Autodesk Inventor part; units mm, degrees
(part 2 of 2)
sketch "Sketch6" plane through (0, 0, 0) normal (0, 0, -1) x (-1, 0, 0)
  line L0 (-4.3025, 26.9125) -> (-4.3025, 11.12) projected
  arc A0 (-4.3025, 26.9125) -> (-7.4775, 30.0875) centre (-7.4775, 26.9125) ccw projected
  line L1 (-8.7475, 30.0875) -> (-7.4775, 30.0875) projected
  arc A1 (-8.7475, 30.0875) -> (-11.9225, 26.9125) centre (-8.7475, 26.9125) ccw projected
  line L2 (-11.9225, 22.4675) -> (-11.9225, 26.9125) projected
  line L3 (-65.8975, 22.4675) -> (-11.9225, 22.4675) projected
  line L4 (-65.8975, 26.9125) -> (-65.8975, 22.4675) projected
  arc A2 (-65.8975, 26.9125) -> (-69.0725, 30.0875) centre (-69.0725, 26.9125) ccw projected
  line L5 (-70.3425, 30.0875) -> (-69.0725, 30.0875) projected
  arc A3 (-70.3425, 30.0875) -> (-73.5175, 26.9125) centre (-70.3425, 26.9125) ccw projected
  line L6 (-73.5175, 8.5836) -> (-73.5175, 26.9125) projected
  line L7 (-76.0575, 6.0436) -> (-73.5175, 8.5836) projected
  line L8 (-76.0575, -27.38) -> (-76.0575, 6.0436) projected
  line L9 (-76.1056, -27.9894) -> (-76.0575, -27.38) projected
  line L10 (-73.5175, -30.5776) -> (-76.1056, -27.9894) projected
  line L11 (-73.5175, -38.4925) -> (-73.5175, -30.5776) projected
  arc A4 (-73.5175, -38.4925) -> (-70.3425, -41.6675) centre (-70.3425, -38.4925) ccw projected
  line L12 (-69.0725, -41.6675) -> (-70.3425, -41.6675) projected
  arc A5 (-69.0725, -41.6675) -> (-65.8975, -38.4925) centre (-69.0725, -38.4925) ccw projected
  line L13 (-65.8975, -34.0475) -> (-65.8975, -38.4925) projected
  line L14 (-11.9225, -34.0475) -> (-65.8975, -34.0475) projected
  line L15 (-11.9225, -38.4925) -> (-11.9225, -34.0475) projected
  arc A6 (-11.9225, -38.4925) -> (-8.7475, -41.6675) centre (-8.7475, -38.4925) ccw projected
  line L16 (-7.4775, -41.6675) -> (-8.7475, -41.6675) projected
  arc A7 (-7.4775, -41.6675) -> (-4.3025, -38.4925) centre (-7.4775, -38.4925) ccw projected
  line L17 (-5.89, -20.285) -> (-5.89, 0) projected
  line L18 (-71.93, -32.46) -> (-5.89, -32.46) projected
  line L19 (-71.93, -29.92) -> (-71.93, -32.46) projected
  line L20 (-74.47, -27.38) -> (-71.93, -29.92) projected
  line L21 (-74.47, 5.386) -> (-74.47, -27.38) projected
  line L22 (-71.93, 7.926) -> (-74.47, 5.386) projected
  line L23 (-71.93, 20.88) -> (-71.93, 7.926) projected
  line L24 (-5.89, 20.88) -> (-71.93, 20.88) projected
  circle A8 centre (-8.1125, -37.8575) radius 2 projected
  circle A9 centre (-69.7075, -37.8575) radius 2 projected
  circle A10 centre (-69.7075, 26.2775) radius 2 projected
  circle A11 centre (-8.1125, 26.2775) radius 2 projected
  line L25 (-23.416, 17.135) -> (-48.816, 17.135) projected
  line L26 (-23.416, 19.545) -> (-23.416, 17.135) projected
  line L27 (-48.816, 19.545) -> (-23.416, 19.545) projected
  line L28 (-48.816, 17.135) -> (-48.816, 19.545) projected
  line L29 (-46.546, 17.34) -> (-46.546, 19.34) projected
  line L30 (-48.546, 17.34) -> (-46.546, 17.34) projected
  line L31 (-48.546, 19.34) -> (-48.546, 17.34) projected
  line L32 (-46.546, 19.34) -> (-48.546, 19.34) projected
  line L33 (-44.006, 17.34) -> (-44.006, 19.34) projected
  line L34 (-46.006, 17.34) -> (-44.006, 17.34) projected
  line L35 (-46.006, 19.34) -> (-46.006, 17.34) projected
  line L36 (-44.006, 19.34) -> (-46.006, 19.34) projected
  line L37 (-41.466, 17.34) -> (-41.466, 19.34) projected
  line L38 (-43.466, 17.34) -> (-41.466, 17.34) projected
  line L39 (-43.466, 19.34) -> (-43.466, 17.34) projected
  line L40 (-41.466, 19.34) -> (-43.466, 19.34) projected
  line L41 (-38.926, 17.34) -> (-38.926, 19.34) projected
  line L42 (-40.926, 17.34) -> (-38.926, 17.34) projected
  line L43 (-40.926, 19.34) -> (-40.926, 17.34) projected
  line L44 (-38.926, 19.34) -> (-40.926, 19.34) projected
  line L45 (-36.386, 17.34) -> (-36.386, 19.34) projected
  line L46 (-38.386, 17.34) -> (-36.386, 17.34) projected
  line L47 (-38.386, 19.34) -> (-38.386, 17.34) projected
  line L48 (-36.386, 19.34) -> (-38.386, 19.34) projected
  line L49 (-33.846, 17.34) -> (-33.846, 19.34) projected
  line L50 (-35.846, 17.34) -> (-33.846, 17.34) projected
  line L51 (-35.846, 19.34) -> (-35.846, 17.34) projected
  line L52 (-33.846, 19.34) -> (-35.846, 19.34) projected
  line L53 (-31.306, 17.34) -> (-31.306, 19.34) projected
  line L54 (-33.306, 17.34) -> (-31.306, 17.34) projected
  line L55 (-33.306, 19.34) -> (-33.306, 17.34) projected
  line L56 (-31.306, 19.34) -> (-33.306, 19.34) projected
  line L57 (-28.766, 17.34) -> (-28.766, 19.34) projected
  line L58 (-30.766, 17.34) -> (-28.766, 17.34) projected
  line L59 (-30.766, 19.34) -> (-30.766, 17.34) projected
  line L60 (-28.766, 19.34) -> (-30.766, 19.34) projected
  line L61 (-28.226, 17.34) -> (-26.226, 17.34) projected
  line L62 (-28.226, 19.34) -> (-28.226, 17.34) projected
  line L63 (-26.226, 19.34) -> (-28.226, 19.34) projected
  line L64 (-26.226, 17.34) -> (-26.226, 19.34) projected
  line L65 (-25.686, 19.34) -> (-25.686, 17.34) projected
  line L66 (-23.686, 19.34) -> (-25.686, 19.34) projected
  line L67 (-23.686, 17.34) -> (-23.686, 19.34) projected
  line L68 (-25.686, 17.34) -> (-23.686, 17.34) projected
  line L69 (-22.41, 16.27) -> (-20.87, 16.27) projected
  arc A12 (-22.41, 16.27) -> (-22.91, 15.77) centre (-22.41, 15.77) ccw projected
  arc A13 (-22.91, 15.77) -> (-23.41, 16.27) centre (-23.41, 15.77) ccw projected
  line L70 (-24.95, 16.27) -> (-23.41, 16.27) projected
  arc A14 (-24.95, 16.27) -> (-25.45, 15.77) centre (-24.95, 15.77) ccw projected
  arc A15 (-25.45, 15.77) -> (-25.95, 16.27) centre (-25.95, 15.77) ccw projected
  line L71 (-27.49, 16.27) -> (-25.95, 16.27) projected
  arc A16 (-27.49, 16.27) -> (-27.99, 15.77) centre (-27.49, 15.77) ccw projected
  line L72 (-27.99, 11.77) -> (-27.99, 15.77) projected
  arc A17 (-27.99, 11.77) -> (-27.49, 11.27) centre (-27.49, 11.77) ccw projected
  line L73 (-25.95, 11.27) -> (-27.49, 11.27) projected
  arc A18 (-25.95, 11.27) -> (-25.45, 11.77) centre (-25.95, 11.77) ccw projected
  arc A19 (-25.45, 11.77) -> (-24.95, 11.27) centre (-24.95, 11.77) ccw projected
  line L74 (-23.41, 11.27) -> (-24.95, 11.27) projected
  arc A20 (-23.41, 11.27) -> (-22.91, 11.77) centre (-23.41, 11.77) ccw projected
  arc A21 (-22.91, 11.77) -> (-22.41, 11.27) centre (-22.41, 11.77) ccw projected
  line L75 (-20.87, 11.27) -> (-22.41, 11.27) projected
  arc A22 (-20.87, 11.27) -> (-20.37, 11.77) centre (-20.87, 11.77) ccw projected
  line L76 (-20.37, 15.77) -> (-20.37, 11.77) projected
  arc A23 (-20.37, 15.77) -> (-20.87, 16.27) centre (-20.87, 15.77) ccw projected
  arc A24 (-24.555, 12.6317) -> (-24.555, 12.3643) centre (-24.178, 12.498) ccw projected
  line L77 (-24.555, 12.875) -> (-24.555, 12.6317) projected
  line L78 (-24.3117, 12.875) -> (-24.555, 12.875) projected
  arc A25 (-24.0443, 12.875) -> (-24.3117, 12.875) centre (-24.178, 12.498) ccw projected
  line L79 (-23.805, 12.875) -> (-24.0443, 12.875) projected
  line L80 (-23.805, 12.6425) -> (-23.805, 12.875) projected
  arc A26 (-23.805, 12.3535) -> (-23.805, 12.6425) centre (-24.178, 12.498) ccw projected
  line L81 (-23.805, 12.125) -> (-23.805, 12.3535) projected
  line L82 (-24.0335, 12.125) -> (-23.805, 12.125) projected
  arc A27 (-24.3225, 12.125) -> (-24.0335, 12.125) centre (-24.178, 12.498) ccw projected
  line L83 (-24.555, 12.125) -> (-24.3225, 12.125) projected
  line L84 (-24.555, 12.3643) -> (-24.555, 12.125) projected
  arc A28 (-24.555, 15.1717) -> (-24.555, 14.9043) centre (-24.178, 15.038) ccw projected
  line L85 (-24.555, 15.415) -> (-24.555, 15.1717) projected
  line L86 (-24.3117, 15.415) -> (-24.555, 15.415) projected
  arc A29 (-24.0443, 15.415) -> (-24.3117, 15.415) centre (-24.178, 15.038) ccw projected
  line L87 (-23.805, 15.415) -> (-24.0443, 15.415) projected
  line L88 (-23.805, 15.1825) -> (-23.805, 15.415) projected
  arc A30 (-23.805, 14.8935) -> (-23.805, 15.1825) centre (-24.178, 15.038) ccw projected
  line L89 (-23.805, 14.665) -> (-23.805, 14.8935) projected
  line L90 (-24.0335, 14.665) -> (-23.805, 14.665) projected
  arc A31 (-24.3225, 14.665) -> (-24.0335, 14.665) centre (-24.178, 15.038) ccw projected
  line L91 (-24.555, 14.665) -> (-24.3225, 14.665) projected
  line L92 (-24.555, 14.9043) -> (-24.555, 14.665) projected
  arc A32 (-27.095, 12.6317) -> (-27.095, 12.3643) centre (-26.718, 12.498) ccw projected
  line L93 (-27.095, 12.875) -> (-27.095, 12.6317) projected
  line L94 (-26.8517, 12.875) -> (-27.095, 12.875) projected
  arc A33 (-26.5843, 12.875) -> (-26.8517, 12.875) centre (-26.718, 12.498) ccw projected
  line L95 (-26.345, 12.875) -> (-26.5843, 12.875) projected
  line L96 (-26.345, 12.6425) -> (-26.345, 12.875) projected
  arc A34 (-26.345, 12.3535) -> (-26.345, 12.6425) centre (-26.718, 12.498) ccw projected
  line L97 (-26.345, 12.125) -> (-26.345, 12.3535) projected
  line L98 (-26.5735, 12.125) -> (-26.345, 12.125) projected
  arc A35 (-26.8625, 12.125) -> (-26.5735, 12.125) centre (-26.718, 12.498) ccw projected
  line L99 (-27.095, 12.125) -> (-26.8625, 12.125) projected
  line L100 (-27.095, 12.3643) -> (-27.095, 12.125) projected
  arc A36 (-27.095, 15.1717) -> (-27.095, 14.9043) centre (-26.718, 15.038) ccw projected
  line L101 (-27.095, 15.415) -> (-27.095, 15.1717) projected
  line L102 (-26.8517, 15.415) -> (-27.095, 15.415) projected
  arc A37 (-26.5843, 15.415) -> (-26.8517, 15.415) centre (-26.718, 15.038) ccw projected
  line L103 (-26.345, 15.415) -> (-26.5843, 15.415) projected
  line L104 (-26.345, 15.1825) -> (-26.345, 15.415) projected
  arc A38 (-26.345, 14.8935) -> (-26.345, 15.1825) centre (-26.718, 15.038) ccw projected
  line L105 (-26.345, 14.665) -> (-26.345, 14.8935) projected
  line L106 (-26.5735, 14.665) -> (-26.345, 14.665) projected
  arc A39 (-26.8625, 14.665) -> (-26.5735, 14.665) centre (-26.718, 15.038) ccw projected
  line L107 (-27.095, 14.665) -> (-26.8625, 14.665) projected
  line L108 (-27.095, 14.9043) -> (-27.095, 14.665) projected
  arc A40 (-22.015, 12.6317) -> (-22.015, 12.3643) centre (-21.638, 12.498) ccw projected
  line L109 (-22.015, 12.875) -> (-22.015, 12.6317) projected
  line L110 (-21.7717, 12.875) -> (-22.015, 12.875) projected
  arc A41 (-21.5043, 12.875) -> (-21.7717, 12.875) centre (-21.638, 12.498) ccw projected
  line L111 (-21.265, 12.875) -> (-21.5043, 12.875) projected
  line L112 (-21.265, 12.6425) -> (-21.265, 12.875) projected
  arc A42 (-21.265, 12.3535) -> (-21.265, 12.6425) centre (-21.638, 12.498) ccw projected
  line L113 (-21.265, 12.125) -> (-21.265, 12.3535) projected
  line L114 (-21.4935, 12.125) -> (-21.265, 12.125) projected
  arc A43 (-21.7825, 12.125) -> (-21.4935, 12.125) centre (-21.638, 12.498) ccw projected
  line L115 (-22.015, 12.125) -> (-21.7825, 12.125) projected
  line L116 (-22.015, 12.3643) -> (-22.015, 12.125) projected
  arc A44 (-22.015, 15.1717) -> (-22.015, 14.9043) centre (-21.638, 15.038) ccw projected
  line L117 (-22.015, 15.415) -> (-22.015, 15.1717) projected
  line L118 (-21.7717, 15.415) -> (-22.015, 15.415) projected
  arc A45 (-21.5043, 15.415) -> (-21.7717, 15.415) centre (-21.638, 15.038) ccw projected
  line L119 (-21.265, 15.415) -> (-21.5043, 15.415) projected
  line L120 (-21.265, 15.1825) -> (-21.265, 15.415) projected
  arc A46 (-21.265, 14.8935) -> (-21.265, 15.1825) centre (-21.638, 15.038) ccw projected
  line L121 (-21.265, 14.665) -> (-21.265, 14.8935) projected
  line L122 (-21.4935, 14.665) -> (-21.265, 14.665) projected
  arc A47 (-21.7825, 14.665) -> (-21.4935, 14.665) centre (-21.638, 15.038) ccw projected
  line L123 (-22.015, 14.665) -> (-21.7825, 14.665) projected
  line L124 (-22.015, 14.9043) -> (-22.015, 14.665) projected
  line L125 (-50.34, 17.135) -> (-70.66, 17.135) projected
  line L126 (-50.34, 19.545) -> (-50.34, 17.135) projected
  line L127 (-70.66, 19.545) -> (-50.34, 19.545) projected
  line L128 (-70.66, 17.135) -> (-70.66, 19.545) projected
  line L129 (-68.39, 17.34) -> (-68.39, 19.34) projected
  line L130 (-70.39, 17.34) -> (-68.39, 17.34) projected
  line L131 (-70.39, 19.34) -> (-70.39, 17.34) projected
  line L132 (-68.39, 19.34) -> (-70.39, 19.34) projected
  line L133 (-65.85, 17.34) -> (-65.85, 19.34) projected
  line L134 (-67.85, 17.34) -> (-65.85, 17.34) projected
  line L135 (-67.85, 19.34) -> (-67.85, 17.34) projected
  line L136 (-65.85, 19.34) -> (-67.85, 19.34) projected
  line L137 (-63.31, 17.34) -> (-63.31, 19.34) projected
  line L138 (-65.31, 17.34) -> (-63.31, 17.34) projected
  line L139 (-65.31, 19.34) -> (-65.31, 17.34) projected
  line L140 (-63.31, 19.34) -> (-65.31, 19.34) projected
  line L141 (-60.77, 17.34) -> (-60.77, 19.34) projected
  line L142 (-62.77, 17.34) -> (-60.77, 17.34) projected
  line L143 (-62.77, 19.34) -> (-62.77, 17.34) projected
  line L144 (-60.77, 19.34) -> (-62.77, 19.34) projected
  line L145 (-58.23, 17.34) -> (-58.23, 19.34) projected
  line L146 (-60.23, 17.34) -> (-58.23, 17.34) projected
  line L147 (-60.23, 19.34) -> (-60.23, 17.34) projected
  line L148 (-58.23, 19.34) -> (-60.23, 19.34) projected
  line L149 (-55.69, 17.34) -> (-55.69, 19.34) projected
  line L150 (-57.69, 17.34) -> (-55.69, 17.34) projected
  line L151 (-57.69, 19.34) -> (-57.69, 17.34) projected
  line L152 (-55.69, 19.34) -> (-57.69, 19.34) projected
  line L153 (-55.15, 17.34) -> (-53.15, 17.34) projected
  line L154 (-55.15, 19.34) -> (-55.15, 17.34) projected
  line L155 (-53.15, 19.34) -> (-55.15, 19.34) projected
  line L156 (-53.15, 17.34) -> (-53.15, 19.34) projected
  line L157 (-52.61, 19.34) -> (-52.61, 17.34) projected
  line L158 (-50.61, 19.34) -> (-52.61, 19.34) projected
  line L159 (-50.61, 17.34) -> (-50.61, 19.34) projected
  line L160 (-52.61, 17.34) -> (-50.61, 17.34) projected
  line L161 (-73.3, -2.8) -> (-73.3, -1.26) projected
  arc A48 (-73.3, -2.8) -> (-72.8, -3.3) centre (-72.8, -2.8) ccw projected
  arc A49 (-72.8, -3.3) -> (-73.3, -3.8) centre (-72.8, -3.8) ccw projected
  line L162 (-73.3, -5.34) -> (-73.3, -3.8) projected
  arc A50 (-73.3, -5.34) -> (-72.8, -5.84) centre (-72.8, -5.34) ccw projected
  arc A51 (-72.8, -5.84) -> (-73.3, -6.34) centre (-72.8, -6.34) ccw projected
  line L163 (-73.3, -7.88) -> (-73.3, -6.34) projected
  arc A52 (-73.3, -7.88) -> (-72.8, -8.38) centre (-72.8, -7.88) ccw projected
  line L164 (-68.8, -8.38) -> (-72.8, -8.38) projected
  arc A53 (-68.8, -8.38) -> (-68.3, -7.88) centre (-68.8, -7.88) ccw projected
  line L165 (-68.3, -6.34) -> (-68.3, -7.88) projected
  arc A54 (-68.3, -6.34) -> (-68.8, -5.84) centre (-68.8, -6.34) ccw projected
  arc A55 (-68.8, -5.84) -> (-68.3, -5.34) centre (-68.8, -5.34) ccw projected
  line L166 (-68.3, -3.8) -> (-68.3, -5.34) projected
  arc A56 (-68.3, -3.8) -> (-68.8, -3.3) centre (-68.8, -3.8) ccw projected
  arc A57 (-68.8, -3.3) -> (-68.3, -2.8) centre (-68.8, -2.8) ccw projected
  line L167 (-68.3, -1.26) -> (-68.3, -2.8) projected
  arc A58 (-68.3, -1.26) -> (-68.8, -0.76) centre (-68.8, -1.26) ccw projected
  line L168 (-72.8, -0.76) -> (-68.8, -0.76) projected
  arc A59 (-72.8, -0.76) -> (-73.3, -1.26) centre (-72.8, -1.26) ccw projected
  arc A60 (-69.905, -4.4308) -> (-69.905, -4.7092) centre (-69.53, -4.57) ccw projected
  line L169 (-69.905, -4.195) -> (-69.905, -4.4308) projected
  line L170 (-69.6692, -4.195) -> (-69.905, -4.195) projected
  arc A61 (-69.3908, -4.195) -> (-69.6692, -4.195) centre (-69.53, -4.57) ccw projected
  line L171 (-69.155, -4.195) -> (-69.3908, -4.195) projected
  line L172 (-69.155, -4.4308) -> (-69.155, -4.195) projected
  arc A62 (-69.155, -4.7092) -> (-69.155, -4.4308) centre (-69.53, -4.57) ccw projected
  line L173 (-69.155, -4.945) -> (-69.155, -4.7092) projected
  line L174 (-69.3908, -4.945) -> (-69.155, -4.945) projected
  arc A63 (-69.6692, -4.945) -> (-69.3908, -4.945) centre (-69.53, -4.57) ccw projected
  line L175 (-69.905, -4.945) -> (-69.6692, -4.945) projected
  line L176 (-69.905, -4.7092) -> (-69.905, -4.945) projected
  arc A64 (-72.445, -4.4308) -> (-72.445, -4.7092) centre (-72.07, -4.57) ccw projected
  line L177 (-72.445, -4.195) -> (-72.445, -4.4308) projected
  line L178 (-72.2092, -4.195) -> (-72.445, -4.195) projected
  arc A65 (-71.9308, -4.195) -> (-72.2092, -4.195) centre (-72.07, -4.57) ccw projected
  line L179 (-71.695, -4.195) -> (-71.9308, -4.195) projected
  line L180 (-71.695, -4.4308) -> (-71.695, -4.195) projected
  arc A66 (-71.695, -4.7092) -> (-71.695, -4.4308) centre (-72.07, -4.57) ccw projected
  line L181 (-71.695, -4.945) -> (-71.695, -4.7092) projected
  line L182 (-71.9308, -4.945) -> (-71.695, -4.945) projected
  arc A67 (-72.2092, -4.945) -> (-71.9308, -4.945) centre (-72.07, -4.57) ccw projected
  line L183 (-72.445, -4.945) -> (-72.2092, -4.945) projected
  line L184 (-72.445, -4.7092) -> (-72.445, -4.945) projected
  arc A68 (-69.905, -6.9708) -> (-69.905, -7.2492) centre (-69.53, -7.11) ccw projected
  line L185 (-69.905, -6.735) -> (-69.905, -6.9708) projected
  line L186 (-69.6692, -6.735) -> (-69.905, -6.735) projected
  arc A69 (-69.3908, -6.735) -> (-69.6692, -6.735) centre (-69.53, -7.11) ccw projected
  line L187 (-69.155, -6.735) -> (-69.3908, -6.735) projected
  line L188 (-69.155, -6.9708) -> (-69.155, -6.735) projected
  arc A70 (-69.155, -7.2492) -> (-69.155, -6.9708) centre (-69.53, -7.11) ccw projected
  line L189 (-69.155, -7.485) -> (-69.155, -7.2492) projected
  line L190 (-69.3908, -7.485) -> (-69.155, -7.485) projected
  arc A71 (-69.6692, -7.485) -> (-69.3908, -7.485) centre (-69.53, -7.11) ccw projected
  line L191 (-69.905, -7.485) -> (-69.6692, -7.485) projected
  line L192 (-69.905, -7.2492) -> (-69.905, -7.485) projected
  line L193 (-72.445, -6.735) -> (-72.445, -7.485) projected
  line L194 (-71.695, -6.735) -> (-72.445, -6.735) projected
  line L195 (-71.695, -7.485) -> (-71.695, -6.735) projected
  line L196 (-72.445, -7.485) -> (-71.695, -7.485) projected
  arc A72 (-69.905, -1.8908) -> (-69.905, -2.1692) centre (-69.53, -2.03) ccw projected
  line L197 (-69.905, -1.655) -> (-69.905, -1.8908) projected
  line L198 (-69.6692, -1.655) -> (-69.905, -1.655) projected
  arc A73 (-69.3908, -1.655) -> (-69.6692, -1.655) centre (-69.53, -2.03) ccw projected
  line L199 (-69.155, -1.655) -> (-69.3908, -1.655) projected
  line L200 (-69.155, -1.8908) -> (-69.155, -1.655) projected
  arc A74 (-69.155, -2.1692) -> (-69.155, -1.8908) centre (-69.53, -2.03) ccw projected
  line L201 (-69.155, -2.405) -> (-69.155, -2.1692) projected
  line L202 (-69.3908, -2.405) -> (-69.155, -2.405) projected
  arc A75 (-69.6692, -2.405) -> (-69.3908, -2.405) centre (-69.53, -2.03) ccw projected
  line L203 (-69.905, -2.405) -> (-69.6692, -2.405) projected
  line L204 (-69.905, -2.1692) -> (-69.905, -2.405) projected
  arc A76 (-72.445, -1.8908) -> (-72.445, -2.1692) centre (-72.07, -2.03) ccw projected
  line L205 (-72.445, -1.655) -> (-72.445, -1.8908) projected
  line L206 (-72.2092, -1.655) -> (-72.445, -1.655) projected
  arc A77 (-71.9308, -1.655) -> (-72.2092, -1.655) centre (-72.07, -2.03) ccw projected
  line L207 (-71.695, -1.655) -> (-71.9308, -1.655) projected
  line L208 (-71.695, -1.8908) -> (-71.695, -1.655) projected
  arc A78 (-71.695, -2.1692) -> (-71.695, -1.8908) centre (-72.07, -2.03) ccw projected
  line L209 (-71.695, -2.405) -> (-71.695, -2.1692) projected
  line L210 (-71.9308, -2.405) -> (-71.695, -2.405) projected
  arc A79 (-72.2092, -2.405) -> (-71.9308, -2.405) centre (-72.07, -2.03) ccw projected
  line L211 (-72.445, -2.405) -> (-72.2092, -2.405) projected
  line L212 (-72.445, -2.1692) -> (-72.445, -2.405) projected
  line L213 (-55.42, -31.125) -> (-70.66, -31.125) projected
  line L214 (-55.42, -28.715) -> (-55.42, -31.125) projected
  line L215 (-70.66, -28.715) -> (-55.42, -28.715) projected
  line L216 (-70.66, -31.125) -> (-70.66, -28.715) projected
  line L217 (-68.39, -30.92) -> (-68.39, -28.92) projected
  line L218 (-70.39, -30.92) -> (-68.39, -30.92) projected
  line L219 (-70.39, -28.92) -> (-70.39, -30.92) projected
  line L220 (-68.39, -28.92) -> (-70.39, -28.92) projected
  line L221 (-65.85, -30.92) -> (-65.85, -28.92) projected
  line L222 (-67.85, -30.92) -> (-65.85, -30.92) projected
  line L223 (-67.85, -28.92) -> (-67.85, -30.92) projected
  line L224 (-65.85, -28.92) -> (-67.85, -28.92) projected
  line L225 (-63.31, -30.92) -> (-63.31, -28.92) projected
  line L226 (-65.31, -30.92) -> (-63.31, -30.92) projected
  line L227 (-65.31, -28.92) -> (-65.31, -30.92) projected
  line L228 (-63.31, -28.92) -> (-65.31, -28.92) projected
  line L229 (-60.77, -30.92) -> (-60.77, -28.92) projected
  line L230 (-62.77, -30.92) -> (-60.77, -30.92) projected
  line L231 (-62.77, -28.92) -> (-62.77, -30.92) projected
  line L232 (-60.77, -28.92) -> (-62.77, -28.92) projected
  line L233 (-60.23, -30.92) -> (-58.23, -30.92) projected
  line L234 (-60.23, -28.92) -> (-60.23, -30.92) projected
  line L235 (-58.23, -28.92) -> (-60.23, -28.92) projected
  line L236 (-58.23, -30.92) -> (-58.23, -28.92) projected
  line L237 (-57.69, -28.92) -> (-57.69, -30.92) projected
  line L238 (-55.69, -28.92) -> (-57.69, -28.92) projected
  line L239 (-55.69, -30.92) -> (-55.69, -28.92) projected
  line L240 (-57.69, -30.92) -> (-55.69, -30.92) projected
  line L241 (-47.53, -28.92) -> (-47.53, -30.92) projected
  line L242 (-32.56, -31.125) -> (-52.88, -31.125) projected
  line L243 (-32.56, -28.715) -> (-32.56, -31.125) projected
  line L244 (-52.88, -28.715) -> (-32.56, -28.715) projected
  line L245 (-52.88, -31.125) -> (-52.88, -28.715) projected
  line L246 (-50.61, -30.92) -> (-50.61, -28.92) projected
  line L247 (-52.61, -30.92) -> (-50.61, -30.92) projected
  line L248 (-52.61, -28.92) -> (-52.61, -30.92) projected
  line L249 (-50.61, -28.92) -> (-52.61, -28.92) projected
  line L250 (-48.07, -30.92) -> (-48.07, -28.92) projected
  line L251 (-50.07, -30.92) -> (-48.07, -30.92) projected
  line L252 (-50.07, -28.92) -> (-50.07, -30.92) projected
  line L253 (-48.07, -28.92) -> (-50.07, -28.92) projected
  line L254 (-45.53, -30.92) -> (-45.53, -28.92) projected
  line L255 (-47.53, -30.92) -> (-45.53, -30.92) projected
  line L256 (-47.53, -28.92) -> (-47.53, -30.92) projected
  line L257 (-45.53, -28.92) -> (-47.53, -28.92) projected
  line L258 (-42.99, -30.92) -> (-42.99, -28.92) projected
  line L259 (-44.99, -30.92) -> (-42.99, -30.92) projected
  line L260 (-44.99, -28.92) -> (-44.99, -30.92) projected
  line L261 (-42.99, -28.92) -> (-44.99, -28.92) projected
  line L262 (-40.45, -30.92) -> (-40.45, -28.92) projected
  line L263 (-42.45, -30.92) -> (-40.45, -30.92) projected
  line L264 (-42.45, -28.92) -> (-42.45, -30.92) projected
  line L265 (-40.45, -28.92) -> (-42.45, -28.92) projected
  line L266 (-37.91, -30.92) -> (-37.91, -28.92) projected
  line L267 (-39.91, -30.92) -> (-37.91, -30.92) projected
  line L268 (-39.91, -28.92) -> (-39.91, -30.92) projected
  line L269 (-37.91, -28.92) -> (-39.91, -28.92) projected
  line L270 (-37.37, -30.92) -> (-35.37, -30.92) projected
  line L271 (-37.37, -28.92) -> (-37.37, -30.92) projected
  line L272 (-35.37, -28.92) -> (-37.37, -28.92) projected
  line L273 (-35.37, -30.92) -> (-35.37, -28.92) projected
  line L274 (-34.83, -28.92) -> (-34.83, -30.92) projected
  line L275 (-32.83, -28.92) -> (-34.83, -28.92) projected
  line L276 (-32.83, -30.92) -> (-32.83, -28.92) projected
  line L277 (-34.83, -30.92) -> (-32.83, -30.92) projected
  circle A80 centre (-12.24, 16.943) radius 1.5 projected
  line L278 (-74.5335, 0.814) -> (-71.93, 0.814) projected
  arc A81 (-71.93, 0.814) -> (-71.93, 5.386) centre (-71.93, 3.1) ccw projected
  line L279 (-71.93, 5.386) -> (-74.5335, 5.386) projected
  line L280 (-74.5335, 5.386) -> (-74.5335, 5.4123) projected
  line L281 (-74.5335, 5.4123) -> (-71.9935, 7.9523) projected
  line L282 (-71.9935, 7.9523) -> (-71.9935, 20.9435) projected
  line L283 (-71.9935, 20.9435) -> (-23.416, 20.9435) projected
  line L284 (-23.416, 20.9435) -> (-23.416, 18.34) projected
  arc A82 (-23.416, 18.34) -> (-18.844, 18.34) centre (-21.13, 18.34) ccw projected
  line L285 (-18.844, 18.34) -> (-18.844, 20.9435) projected
  line L286 (-18.844, 20.9435) -> (-5.8265, 20.9435) projected
  line L287 (-5.8265, 20.9435) -> (-5.8265, 11.12) projected
  line L288 (-5.8265, 11.12) -> (-5.89, 11.12) projected
  line L289 (-5.89, 11.12) -> (-5.89, 0) projected
  line L290 (-5.89, 0) -> (-5.8265, 0) projected
  line L291 (-5.8265, -29.285) -> (-5.8265, -32.5235) projected
  line L292 (-5.8265, -20.285) -> (-5.89, -20.285) projected
  line L293 (-5.89, -20.285) -> (-5.89, -29.285) projected
  line L294 (-5.89, -29.285) -> (-5.8265, -29.285) projected
  line L295 (-5.8265, 0) -> (-5.8265, -20.285) projected
  line L296 (-5.8265, -32.5235) -> (-71.9935, -32.5235) projected
  line L297 (-71.9935, -32.5235) -> (-71.9935, -29.9463) projected
  line L298 (-71.9935, -29.9463) -> (-74.5335, -27.4063) projected
  line L299 (-74.5335, -27.4063) -> (-74.5335, -27.126) projected
  line L300 (-74.5335, -27.126) -> (-71.93, -27.126) projected
  arc A83 (-71.93, -27.126) -> (-71.93, -22.554) centre (-71.93, -24.84) ccw projected
  line L301 (-71.93, -22.554) -> (-74.5335, -22.554) projected
  line L302 (-74.5335, -22.554) -> (-74.5335, 0.814) projected
  line L303 (-22.146, -29.92) -> (-22.146, -32.46) projected
  line L304 (-22.146, -32.46) -> (-17.574, -32.46) projected
  line L305 (-17.574, -32.46) -> (-17.574, -29.92) projected
  arc A84 (-17.574, -29.92) -> (-22.146, -29.92) centre (-19.86, -29.92) ccw projected
  line L306 (-5.89, 11.12) -> (-4.3025, 11.12) projected
  line L307 (-4.3025, -29.285) -> (-4.3025, -38.4925) projected
  line L308 (-4.3025, -29.285) -> (-5.89, -29.285) projected
  line L309 (-5.89, -32.46) -> (-5.89, -29.285) projected
  line L310 (-5.89, 11.12) -> (-5.89, 20.88) projected
  line L311 (-4.3025, 0) -> (-5.89, 0) projected
  line L312 (-5.89, -20.285) -> (-4.3025, -20.285) projected
  line L313 (-4.3025, 0) -> (-4.3025, -20.285) projected
  point P0 (0, 0)
sketch "Sketch8" plane through (0, 0, 21.35) normal (0, 0, 1) x (1, 0, 0)
  line L0 (15.48, 11.58) -> (0.1, 11.58) projected
  line L1 (4.3025, 20.88) -> (4.3025, -32.46) projected
  line L2 (5.89, 11.12) -> (5.89, 0) projected
  line L3 (0.1, -0.46) -> (15.48, -0.46) projected
  line L4 (5.8265, 11.12) -> (5.8265, 20.9435) projected
  line L5 (5.8265, -20.285) -> (5.8265, 0) projected
  line L6 (5.8265, 11.12) -> (4.3025, 11.12)
  line L7 (4.3025, 11.12) -> (4.3025, -0.46)
  line L8 (4.3025, -0.46) -> (5.8265, -0.46)
  line L9 (5.8265, -0.46) -> (5.8265, 11.12)
  line L10 (4.3025, 11.12) -> (5.8265, 11.12)
  line L11 (5.8265, 11.12) -> (5.8265, 11.58)
  line L12 (5.8265, 11.58) -> (4.3025, 11.58)
  line L13 (4.3025, 11.58) -> (4.3025, 11.12)
  point P0 (0, 0)
  point P1 (4.3025, 11.58)
  point P2 (5.8265, -0.46)
  constraints: 16 end point, 4 parallel, 4 point on line, 2 horizontal, 2 perpendicular
extrude "Extrusion10" cut sketch "Sketch8" against normal up to surface (15 mm away)
sketch "Sketch9" plane through (0, 0, 6.35) normal (0, 0, 1) x (1, 0, 0)
  line L0 (4.3025, 11.12) -> (5.89, 11.12) projected
  line L1 (4.3025, 11.12) -> (5.89, 11.12)
  line L2 (5.89, 11.12) -> (5.89, 0)
  line L3 (5.89, 0) -> (4.3025, 0)
  line L4 (4.3025, 0) -> (4.3025, 11.12)
  line L5 (4.3025, -20.285) -> (5.8265, -20.285) projected
  line L6 (5.89, -29.285) -> (5.8265, -29.285) projected
  line L7 (4.3025, -20.285) -> (5.89, -20.285)
  line L8 (5.89, -20.285) -> (5.89, -29.285)
  line L9 (5.89, -29.285) -> (4.3025, -29.285)
  line L10 (4.3025, -29.285) -> (4.3025, -20.285)
  point P0 (0, 0)
  constraints: 16 end point, 4 parallel, 2 horizontal, 2 perpendicular
extrude "Extrusion11" add sketch "Sketch9" against normal blind 6.35
sketch "Sketch10" plane through (0, 0, 6.35) normal (0, 0, 1) x (1, 0, 0)
  line L0 (4.3025, 11.58) -> (5.8265, 11.58) projected
  line L1 (5.8265, -0.46) -> (4.3025, -0.46) projected
  line L2 (4.3025, 11.58) -> (5.8265, 11.58)
  line L3 (5.8265, 11.58) -> (5.8265, -0.46)
  line L4 (5.8265, -0.46) -> (4.3025, -0.46)
  line L5 (4.3025, -0.46) -> (4.3025, 11.58)
  line L6 (4.3025, -20.285) -> (5.8265, -20.285) projected
  line L7 (5.8265, -29.285) -> (4.3025, -29.285) projected
  line L8 (4.3025, -20.285) -> (5.8265, -20.285)
  line L9 (5.8265, -20.285) -> (5.8265, -29.285)
  line L10 (5.8265, -29.285) -> (4.3025, -29.285)
  line L11 (4.3025, -29.285) -> (4.3025, -20.285)
  point P0 (0, 0)
  constraints: 16 end point, 4 parallel, 2 horizontal, 2 perpendicular
extrude "Extrusion12" add sketch "Sketch10" along normal blind 3.5
sketch "Sketch11" plane through (0, 0, 21.35) normal (0, 0, 1) x (1, 0, 0)
  line L0 (5.8265, -20.285) -> (5.8265, -0.46) projected
  line L1 (4.3025, -0.46) -> (4.3025, -20.285) projected
  line L2 (5.8265, -20.285) -> (4.3025, -20.285)
  line L3 (4.3025, -20.285) -> (4.3025, -19.3376)
  line L4 (4.3025, -19.3376) -> (5.8265, -19.3376)
  line L5 (5.8265, -19.3376) -> (5.8265, -20.285)
  point P0 (0, 0)
  constraints: 8 end point, 2 parallel, 1 horizontal, 1 perpendicular, 1 point on line
extrude "Extrusion13" cut sketch "Sketch11" against normal up to surface (11.5 mm away)
sketch "Sketch12" plane through (0, 0, 21.35) normal (0, 0, 1) x (1, 0, 0)
  line L0 (32.56, -31.125) -> (52.88, -31.125) projected
  line L1 (55.42, -31.125) -> (70.66, -31.125) projected
  line L2 (70.66, 19.545) -> (50.34, 19.545) projected
  line L3 (48.816, 19.545) -> (23.416, 19.545) projected
  line L4 (65.8975, 22.4675) -> (73.5175, 22.4675) projected
  line L5 (23.416, 19.545) -> (70.66, 19.545)
  line L6 (70.66, 19.545) -> (70.66, 22.4675)
  line L7 (70.66, 22.4675) -> (23.416, 22.4675)
  line L8 (23.416, 22.4675) -> (23.416, 19.545)
  line L9 (4.3025, -34.0475) -> (73.5175, -34.0475) projected
  line L10 (70.66, -31.125) -> (32.56, -31.125)
  line L11 (32.56, -31.125) -> (32.56, -34.0475)
  line L12 (32.56, -34.0475) -> (70.66, -34.0475)
  line L13 (70.66, -34.0475) -> (70.66, -31.125)
  point P0 (0, 0)
  constraints: 16 end point, 4 parallel, 2 horizontal, 2 perpendicular, 2 point on line
extrude "Extrusion14" cut sketch "Sketch12" against normal blind 11.43
sketch "Sketch13" plane through (0, 0, 21.35) normal (0, 0, 1) x (1, 0, 0)
  line L0 (73.5175, 22.4675) -> (70.66, 22.4675) projected
  line L1 (73.5175, 22.4675) -> (71.0283, 22.4675)
  line L2 (70.66, -32.5235) -> (70.66, -34.0475) projected
  line L3 (71.0283, 22.4675) -> (70.66, 22.4675)
  line L4 (70.66, 22.4675) -> (70.66, -34.0475)
  line L5 (70.66, -34.0475) -> (71.0283, -34.0475)
  line L6 (71.0283, -34.0475) -> (71.0283, 22.4675)
  point P0 (0, 0)
  dimension "d54" = 2.4892
  constraints: 10 end point, 2 parallel, 1 horizontal, 1 perpendicular, 1 point on line
  measures "d54" distance of L0.start L1.end
extrude "Extrusion15" cut sketch "Sketch13" against normal up to surface (11.43 mm away)
body "Solid1"
